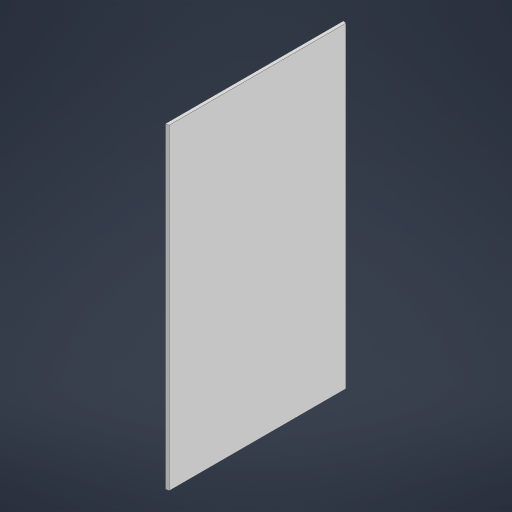
# Autodesk Inventor part: Battery_platform
Saved by Autodesk Inventor 2024 (Build 280153000, 153)
## iProperties
Created: 2024-02-29
Part Number: Battery_platform
Material: Generic
Document SubType Name: Modeling
Designer: calvi
Density: 1 g/cm^3
Appearance: Default
Author: calvi
Autodesk Inventor part; units mm, degrees
ref_plane "YZ Plane" through (0, 0, 0) normal (1, 0, 0) x (0, 1, 0)
ref_plane "XZ Plane" through (0, 0, 0) normal (0, 1, 0) x (-1, 0, 0)
ref_plane "XY Plane" through (0, 0, 0) normal (0, 0, 1) x (1, 0, 0)
sketch "Sketch1" plane through (0, 0, 0) normal (0, 1, 0) x (-1, 0, 0)
  line L0 (0, 0) -> (25.4, 0)
  line L1 (25.4, 0) -> (25.4, -120.904)
  line L2 (25.4, -120.904) -> (0, -120.904)
  line L3 (0, -120.904) -> (0, 0)
  arc A0 (25.4, 25.4) -> (0, 0) centre (25.4, 0) ccw
  arc A1 (0, -120.904) -> (25.4, -146.304) centre (25.4, -120.904) ccw
  line L4 (25.4, 0) -> (25.4, 25.4)
  line L5 (25.4, -120.904) -> (25.4, -146.304)
  dimension "d0" = 25.4
  dimension "d1" = 120.904
  constraints: 12 end point, 5 point on circle, 2 centre point, 2 coincident, 2 parallel, 2 point on line, 1 horizontal, 1 perpendicular, 1 vertical
  measures "d0" distance of L1.end L2.end
  measures "d1" distance of L0.end L1.end
extrude "Extrusion1" add sketch "Sketch1" along normal blind 304.8
sketch "Sketch3" plane through (0, 304.8, 0) normal (0, 1, 0) x (1, 0, 0)
  arc A0 (-25.4, -25.4) -> (0, 0) centre (-25.4, 0) ccw projected
  line L0 (-25.4, -25.4) -> (-22.352, -25.4)
  line L1 (-22.352, -25.4) -> (-22.352, 146.304)
  line L2 (-22.352, 146.304) -> (-25.4, 146.304)
  line L3 (-25.4, 146.304) -> (-25.4, -25.4)
  line L4 (-22.352, -25.4) -> (0, -25.4)
  line L5 (0, -25.4) -> (0, 146.304)
  line L6 (0, 146.304) -> (-22.352, 146.304)
  line L7 (-22.352, 146.304) -> (-22.352, -25.4)
  line L8 (0, 0) -> (0, 120.904) projected
  line L9 (-22.352, -25.4) -> (-19.304, -25.4)
  line L10 (-19.304, -25.4) -> (-19.304, 146.304)
  line L11 (-19.304, 146.304) -> (-22.352, 146.304)
  line L12 (-22.352, 146.304) -> (-22.352, -25.4)
  point P0 (-19.304, -24.6576)
  point P1 (0, 0)
  point P2 (-22.352, -25.2165)
  dimension "d4" = 3.048
  dimension "d5" = 171.704
  dimension "d6" = 0
  dimension "d7" = 171.704
  dimension "d8" = 3.048
  constraints: 24 end point, 6 parallel, 3 horizontal, 3 perpendicular, 1 point on line
  measures "d4" distance of L2.end L1.end
  measures "d5" distance of L1.end L0.end
  measures "d6" distance between parallel lines of L8 L5
  measures "d7" distance between parallel lines of L6 L4
  measures "d8" distance of L11.end L10.end
extrude "Extrusion2" cut sketch "Sketch3" against normal through all contours L3 L2 L1 A0 | L10 L6 L5 A0
body "Solid1"
